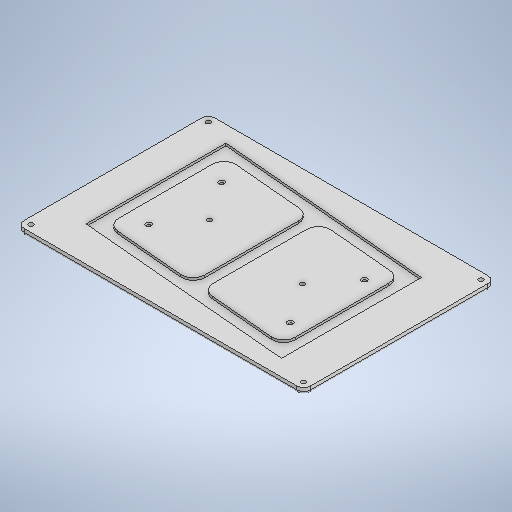
# Autodesk Inventor part: BackPlate
Saved by Autodesk Inventor 2025.2 (Build 292293000, 293)
## iProperties
Created: 2026-02-06
Part Number: BackPlate
Material: Generic
Document SubType Name: Modeling
Designer: Joefi
Density: 1 g/cm^3
Appearance: Default
Mass: 233.651 g
Surface Area: 902.919 cm^2
Volume: 233.651 cm^3
Author: Joefi
Autodesk Inventor part; units mm, degrees
ref_plane "YZ Plane" through (0, 0, 0) normal (1, 0, 0) x (0, 1, 0)
ref_plane "XZ Plane" through (0, 0, 0) normal (0, 1, 0) x (-1, 0, 0)
ref_plane "XY Plane" through (0, 0, 0) normal (0, 0, 1) x (1, 0, 0)
sketch "Sketch1" plane through (0, 0, 0) normal (0, 1, 0) x (-1, 0, 0)
  circle A0 centre (119, 77.3333) radius 2
  circle A1 centre (-119, -77.3333) radius 2
  arc A2 (119, -83.3333) -> (125, -77.3333) centre (119, -77.3333) ccw
  line L0 (125, -77.3333) -> (125, 77.3333)
  arc A3 (125, 77.3333) -> (119, 83.3333) centre (119, 77.3333) ccw
  line L1 (119, 83.3333) -> (-119, 83.3333)
  arc A4 (-119, 83.3333) -> (-125, 77.3333) centre (-119, 77.3333) ccw
  line L2 (-125, 77.3333) -> (-125, -77.3333)
  arc A5 (-125, -77.3333) -> (-119, -83.3333) centre (-119, -77.3333) ccw
  line L3 (-119, -83.3333) -> (119, -83.3333)
  line L4 (119, 71.3333) -> (119, -71.3333)
  arc A6 (119, -71.3333) -> (113, -77.3333) centre (119, -77.3333) ccw
  line L5 (113, -77.3333) -> (-113, -77.3333)
  arc A7 (-113, -77.3333) -> (-119, -71.3333) centre (-119, -77.3333) ccw
  line L6 (-119, -71.3333) -> (-119, 71.3333)
  arc A8 (-119, 71.3333) -> (-113, 77.3333) centre (-119, 77.3333) ccw
  line L7 (-113, 77.3333) -> (113, 77.3333)
  arc A9 (113, 77.3333) -> (119, 71.3333) centre (119, 77.3333) ccw
  circle A10 centre (-119, 77.3333) radius 2
  circle A11 centre (119, -77.3333) radius 2
  point P0 (0, 0)
  point P1 (0, 0)
  dimension "d20" = 4
  dimension "d21" = 4
  dimension "d22" = 4
  dimension "d23" = 4
  constraints: 16 end point, 16 point on circle, 12 centre point, 4 horizontal, 4 vertical, 38 other
  measures "d20" diameter of A1
  measures "d21" diameter of A10
  measures "d22" diameter of A0
  measures "d23" diameter of A11
extrude "Extrusion1" add sketch "Sketch1" along normal blind 6 contours L3 A5 L2 A4 L1 A3 L0 A2 | L4 A6 L5 A7 L6 A8 L7 A9
sketch "Sketch4" plane through (0, 6, 0) normal (0, 1, 0) x (1, 0, 0)
  line L0 (-102.1195, -45.2048) -> (-102.1195, -30.4721) construction
  line L1 (-75.2032, -31.8232) -> (-102.1195, -29.4683) construction
  line L2 (-0.5, -66.4658) -> (-89.7961, -58.6534) construction
  line L3 (-73.7032, -31.4525) -> (-15, -36.5884) construction
  line L4 (-102.1195, -30.4721) -> (-15.8441, -38.0202) construction
  line L5 (-73.7032, 44.3489) -> (-73.7032, -31.4525) construction
  line L6 (-102.1195, -29.4683) -> (-102.1195, 47.3369) construction
  line L7 (-103.1195, 60.7112) -> (-103.1195, -45.2048) construction
  line L8 (-13.5, -39.8412) -> (-13.5, 41.8938) construction
  line L9 (-15, -36.5884) -> (-15, 39.213) construction
  line L10 (-16.1525, 40.8196) -> (-102.1195, 48.3407) construction
  line L11 (-15, 39.213) -> (-73.7032, 44.3489) construction
  line L12 (-13.5, 41.8938) -> (0.1542, 54.4056) construction
  line L13 (-0.5, 55.1624) -> (-16.1525, 40.8196) construction
  line L14 (-87.4429, 74.1598) -> (-0.5, 66.5533) construction
  line L15 (-0.5, 66.5533) -> (-0.5, 55.1624) construction
  line L16 (0.5, 54.7653) -> (0.5, 66.4658) construction
  line L17 (0.1542, 54.4056) -> (13.5, 39.8412) construction
  line L18 (15.8441, 38.0202) -> (0.5, 54.7653) construction
  line L19 (-75.2032, 44.982) -> (-75.2032, -31.8232) construction
  line L20 (0.5, -55.1624) -> (16.1525, -40.8196) construction
  line L21 (0.5, -66.5533) -> (0.5, -55.1624) construction
  line L22 (-0.5, -54.7653) -> (-0.5, -66.4658) construction
  line L23 (13.5, -41.8938) -> (-0.1542, -54.4056) construction
  line L24 (-0.1542, -54.4056) -> (-13.5, -39.8412) construction
  line L25 (-15.8441, -38.0202) -> (-0.5, -54.7653) construction
  line L26 (-89.8832, -59.6496) -> (87.3557, -75.156) construction
  line L27 (89.8832, 59.6496) -> (-87.3557, 75.156) construction
  line L28 (102.1195, 45.2048) -> (102.1195, 30.4721) construction
  arc A0 (102.1195, 45.2048) -> (89.7961, 58.6534) centre (88.6195, 45.2048) ccw construction
  arc A1 (103.1195, 45.2048) -> (89.8832, 59.6496) centre (88.6195, 45.2048) ccw construction
  line L29 (75.2032, 31.8232) -> (102.1195, 29.4683) construction
  line L30 (14.5, -39.6712) -> (14.5, 37.134) construction
  line L31 (13.5, 39.8412) -> (13.5, -41.8938) construction
  line L32 (14.5, 37.134) -> (74.2032, 31.9107) construction
  line L33 (74.2032, -44.8945) -> (14.5, -39.6712) construction
  line L34 (75.2032, -44.982) -> (75.2032, 31.8232) construction
  line L35 (0.5, 66.4658) -> (89.7961, 58.6534) construction
  line L36 (87.4429, -74.1598) -> (0.5, -66.5533) construction
  line L37 (102.1195, 30.4721) -> (15.8441, 38.0202) construction
  line L38 (16.1525, -40.8196) -> (102.1195, -48.3407) construction
  line L39 (103.1195, -60.7112) -> (103.1195, 45.2048) construction
  line L40 (102.1195, -47.3369) -> (75.2032, -44.982) construction
  line L41 (102.1195, -48.3407) -> (102.1195, -60.7112) construction
  arc A2 (87.4429, -74.1598) -> (102.1195, -60.7112) centre (88.6195, -60.7112) ccw construction
  arc A3 (87.3557, -75.156) -> (103.1195, -60.7112) centre (88.6195, -60.7112) ccw construction
  line L42 (102.1195, 29.4683) -> (102.1195, -47.3369) construction
  line L43 (74.2032, 31.9107) -> (74.2032, -44.8945) construction
  arc A4 (-102.1195, -45.2048) -> (-89.7961, -58.6534) centre (-88.6195, -45.2048) ccw construction
  arc A5 (-103.1195, -45.2048) -> (-89.8832, -59.6496) centre (-88.6195, -45.2048) ccw construction
  arc A6 (-87.3557, 75.156) -> (-103.1195, 60.7112) centre (-88.6195, 60.7112) ccw construction
  arc A7 (-87.4429, 74.1598) -> (-102.1195, 60.7112) centre (-88.6195, 60.7112) ccw construction
  line L44 (-102.1195, 48.3407) -> (-102.1195, 60.7112) construction
  line L45 (-102.1195, 47.3369) -> (-75.2032, 44.982) construction
  line L46 (5, -48) -> (-5, -48)
  line L47 (-5, -48) -> (-5, 48)
  line L48 (-5, 48) -> (5, 48)
  line L49 (5, 48) -> (5, -48)
  line L50 (5, -48) -> (-5, 48) construction
  line L51 (-5, -48) -> (5, 48) construction
  line L52 (-90.4115, -45.6034) -> (-90.4115, 61.1094) construction
  line L53 (-90.4115, 63.7374) -> (86.4661, 48.2626) construction
  line L54 (86.4661, 45.2048) -> (86.4661, -60.7112) construction
  line L55 (86.4661, -63.7374) -> (-90.4115, -48.2626) construction
  line L56 (91.4661, -55.7532) -> (86.4661, -55.7532)
  line L57 (81.4661, -55.7532) -> (81.4661, 40.2468)
  line L58 (86.4661, 40.2468) -> (91.4661, 40.2468)
  line L59 (91.4661, 40.2468) -> (91.4661, -55.7532)
  line L60 (91.4661, -55.7532) -> (81.4661, 40.2468) construction
  line L61 (81.4661, -55.7532) -> (91.4661, 40.2468) construction
  line L62 (-90.4115, -40.247) -> (-95.4115, -40.247)
  line L63 (-95.4115, -40.247) -> (-95.4115, 55.753)
  line L64 (-95.4115, 55.753) -> (-90.4115, 55.753)
  line L65 (-85.4115, 55.753) -> (-85.4115, -40.247)
  line L66 (-85.4115, -40.247) -> (-95.4115, 55.753) construction
  line L67 (-95.4115, -40.247) -> (-85.4115, 55.753) construction
  line L68 (95.2186, -69.5222) -> (-100.0356, -52.4397)
  line L69 (-100.0356, -52.4397) -> (-99.164, -42.4778)
  line L70 (96.0902, -59.5603) -> (95.2186, -69.5222)
  line L71 (95.2186, -69.5222) -> (-99.164, -42.4778) construction
  line L72 (-100.0356, -52.4397) -> (96.0902, -59.5603) construction
  line L73 (-100.0356, 59.5603) -> (-99.164, 69.5222)
  line L74 (-99.164, 69.5222) -> (96.0902, 52.4397)
  line L75 (96.0902, 52.4397) -> (95.2186, 42.4778)
  line L76 (95.2186, 42.4778) -> (-99.164, 69.5222) construction
  line L77 (-100.0356, 59.5603) -> (96.0902, 52.4397) construction
  line L78 (81.4661, 40.2468) -> (81.4661, 43.681)
  line L79 (91.4661, -55.7532) -> (91.4661, -59.1557)
  line L80 (5, -48) -> (5, -51.5909)
  line L81 (-5, 48) -> (-5, 51.2458)
  line L82 (-95.4115, 55.753) -> (-95.4115, 59.1557)
  line L83 (-85.4115, -40.247) -> (-85.4115, -43.681)
  line L84 (5, 48) -> (5, 50.3709)
  line L85 (-5, -48) -> (-5, -50.716)
  line L86 (-95.4115, -40.247) -> (-95.4115, -42.8061)
  line L87 (-85.4115, 55.753) -> (-85.4115, 58.2808)
  line L88 (91.4661, 40.2468) -> (91.4661, 42.8061)
  line L89 (81.4661, -55.7532) -> (81.4661, -58.2808)
  line L90 (-90.4115, 58.7183) -> (-100.0356, 59.5603)
  line L91 (-99.164, -42.4778) -> (-90.4115, -43.2435)
  line L92 (86.4661, -58.7183) -> (96.0902, -59.5603)
  line L93 (95.2186, 42.4778) -> (86.4661, 43.2435)
  line L94 (81.4661, 43.681) -> (3.7512, 50.4801)
  line L95 (-3.4428, 51.1095) -> (-85.4115, 58.2808)
  line L96 (-85.4115, -43.681) -> (-3.4074, -50.8554)
  line L97 (3.0989, -51.4246) -> (81.4661, -58.2808)
  line L98 (-95.4115, -42.8061) -> (-95.4115, -52.8443)
  line L99 (-95.4115, 59.1557) -> (-95.4115, 69.1939)
  line L100 (91.4661, 42.8061) -> (91.4661, 52.8443)
  line L101 (91.4661, -59.1557) -> (91.4661, -69.1939)
  point P0 (0, 0)
  point P1 (0, 0)
  point P2 (86.4661, -7.7532)
  point P3 (-90.4115, 7.753)
  point P4 (-1.9727, -56)
  point P5 (-1.9727, 56)
  point P6 (-1.9727, 56)
  dimension "d2" = 10
  dimension "d3" = 96
  dimension "d4" = 10
  dimension "d5" = 96
  dimension "d6" = 10
  dimension "d7" = 96
  dimension "d8" = 10
  dimension "d11" = 196
  dimension "d12" = 10
  dimension "d13" = 196
  dimension "d48" = 56
  dimension "d49" = 56
  constraints: 200 end point, 32 parallel, 25 vertical, 19 point on line, 16 point on circle, 13 midpoint, 8 centre point, 7 perpendicular, 3 horizontal, 112 other
  measures "d2" distance of L47.end L48.end
  measures "d3" distance of L46.end L47.end
  measures "d4" distance of L57.end L58.end
  measures "d5" distance of L57.start L57.end
  measures "d6" distance of L63.end L65.start
  measures "d7" distance of L62.end L63.end
  measures "d8" distance of L68.end L69.end
  measures "d11" distance of L68.start L68.end
  measures "d12" distance of L73.start L73.end
  measures "d13" distance of L73.end L74.end
  measures "d48" vertical distance of point (0, 0) point (-1.973, -56)
  measures "d49" vertical distance of point (-1.973, 56) point (0, 0)
extrude "Extrusion2" cut sketch "Sketch4" against normal blind 2 contours L46 L47 L48 L49 | L59 L79 L101 L68 L98 L86 L63 L82 L99 L74 L100 L88
sketch "Sketch5" plane through (0, 0, 0) normal (0, -1, 0) x (1, 0, 0)
  circle A0 centre (119, 77.3333) radius 2.45
  circle A1 centre (-119, -77.3333) radius 2.45
  arc A2 (119, -83.3333) -> (125, -77.3333) centre (119, -77.3333) ccw
  line L0 (125, -77.3333) -> (125, 77.3333)
  arc A3 (125, 77.3333) -> (119, 83.3333) centre (119, 77.3333) ccw
  line L1 (119, 83.3333) -> (-119, 83.3333)
  arc A4 (-119, 83.3333) -> (-125, 77.3333) centre (-119, 77.3333) ccw
  line L2 (-125, 77.3333) -> (-125, -77.3333)
  arc A5 (-125, -77.3333) -> (-119, -83.3333) centre (-119, -77.3333) ccw
  line L3 (-119, -83.3333) -> (119, -83.3333)
  line L4 (119, 71.3333) -> (119, -71.3333)
  arc A6 (119, -71.3333) -> (113, -77.3333) centre (119, -77.3333) ccw
  line L5 (113, -77.3333) -> (-113, -77.3333)
  arc A7 (-113, -77.3333) -> (-119, -71.3333) centre (-119, -77.3333) ccw
  line L6 (-119, -71.3333) -> (-119, 71.3333)
  arc A8 (-119, 71.3333) -> (-113, 77.3333) centre (-119, 77.3333) ccw
  line L7 (-113, 77.3333) -> (113, 77.3333)
  arc A9 (113, 77.3333) -> (119, 71.3333) centre (119, 77.3333) ccw
  circle A10 centre (-119, 77.3333) radius 2.45
  circle A11 centre (119, -77.3333) radius 2.45
  circle A12 centre (-44.3516, -3.8803) radius 6
  circle A13 centre (44.3516, 3.8803) radius 6
  circle A14 centre (-44.3516, -3.8803) radius 2
  circle A15 centre (44.3516, 3.8803) radius 2
  point P0 (0, 0)
  point P1 (0, 0)
  dimension "d16" = 4
  dimension "d17" = 4
  constraints: 16 centre point, 16 end point, 16 point on circle, 2 coincident
  measures "d16" diameter of A14
  measures "d17" diameter of A15
extrude "Extrusion3" cut sketch "Sketch5" against normal through all contours A14 | A15
chamfer "Chamfer1" distance 1 angle 45 6 edges at (-117, 0, -77.3333) (-46.3516, 0, -3.8803) (-117, 0, 77.3333) (42.3516, 0, 3.8803) (121, 0, 77.3333) (121, 0, -77.3333)
fillet "Fillet1" radius 3 8 edges at (123.2426, 0, -81.576) (0, 0, -83.3333) (-123.2426, 0, -81.576) (-125, 0, 0) (-123.2426, 0, 81.576) (0, 0, 83.3333) (123.2426, 0, 81.576) (125, 0, 0)
sketch "Sketch6" plane through (0, 6, 0) normal (0, 1, 0) x (1, 0, 0)
  arc A0 (-87.3557, 75.156) -> (-103.1195, 60.7112) centre (-88.6195, 60.7112) ccw construction
  arc A1 (-87.4429, 74.1598) -> (-102.1195, 60.7112) centre (-88.6195, 60.7112) ccw construction
  line L0 (-102.1195, 48.3407) -> (-102.1195, 60.7112) construction
  line L1 (-16.1525, 40.8196) -> (-102.1195, 48.3407) construction
  line L2 (-15, 39.213) -> (-73.7032, 44.3489) construction
  line L3 (-87.4429, 74.1598) -> (-0.5, 66.5533) construction
  line L4 (89.8832, 59.6496) -> (-87.3557, 75.156) construction
  line L5 (-0.5, 55.1624) -> (-16.1525, 40.8196) construction
  line L6 (-0.5, 66.5533) -> (-0.5, 55.1624) construction
  line L7 (0.5, 54.7653) -> (0.5, 66.4658) construction
  line L8 (0.1542, 54.4056) -> (13.5, 39.8412) construction
  line L9 (15.8441, 38.0202) -> (0.5, 54.7653) construction
  line L10 (-13.5, 41.8938) -> (0.1542, 54.4056) construction
  line L11 (-0.5, -66.4658) -> (-89.7961, -58.6534) construction
  line L12 (-15.8441, -38.0202) -> (-0.5, -54.7653) construction
  line L13 (-0.1542, -54.4056) -> (-13.5, -39.8412) construction
  line L14 (13.5, -41.8938) -> (-0.1542, -54.4056) construction
  arc A2 (-102.1195, -45.2048) -> (-89.7961, -58.6534) centre (-88.6195, -45.2048) ccw construction
  arc A3 (-103.1195, -45.2048) -> (-89.8832, -59.6496) centre (-88.6195, -45.2048) ccw construction
  line L15 (-0.5, -54.7653) -> (-0.5, -66.4658) construction
  line L16 (0.5, -66.5533) -> (0.5, -55.1624) construction
  line L17 (-89.8832, -59.6496) -> (87.3557, -75.156) construction
  line L18 (0.5, -55.1624) -> (16.1525, -40.8196) construction
  line L19 (14.5, -39.6712) -> (14.5, 37.134) construction
  line L20 (13.5, 39.8412) -> (13.5, -41.8938) construction
  line L21 (74.2032, 31.9107) -> (74.2032, -44.8945) construction
  line L22 (75.2032, -44.982) -> (75.2032, 31.8232) construction
  line L23 (103.1195, -60.7112) -> (103.1195, 45.2048) construction
  line L24 (102.1195, 29.4683) -> (102.1195, -47.3369) construction
  line L25 (102.1195, -47.3369) -> (75.2032, -44.982) construction
  line L26 (74.2032, -44.8945) -> (14.5, -39.6712) construction
  line L27 (16.1525, -40.8196) -> (102.1195, -48.3407) construction
  line L28 (87.4429, -74.1598) -> (0.5, -66.5533) construction
  line L29 (102.1195, -48.3407) -> (102.1195, -60.7112) construction
  line L30 (14.5, 37.134) -> (74.2032, 31.9107) construction
  line L31 (102.1195, 30.4721) -> (15.8441, 38.0202) construction
  line L32 (0.5, 66.4658) -> (89.7961, 58.6534) construction
  line L33 (75.2032, 31.8232) -> (102.1195, 29.4683) construction
  line L34 (102.1195, 45.2048) -> (102.1195, 30.4721) construction
  arc A4 (102.1195, 45.2048) -> (89.7961, 58.6534) centre (88.6195, 45.2048) ccw construction
  arc A5 (103.1195, 45.2048) -> (89.8832, 59.6496) centre (88.6195, 45.2048) ccw construction
  line L35 (-102.1195, -45.2048) -> (-102.1195, -30.4721) construction
  line L36 (-75.2032, -31.8232) -> (-102.1195, -29.4683) construction
  line L37 (-73.7032, -31.4525) -> (-15, -36.5884) construction
  line L38 (-102.1195, -30.4721) -> (-15.8441, -38.0202) construction
  line L39 (-15, -36.5884) -> (-15, 39.213) construction
  line L40 (-13.5, -39.8412) -> (-13.5, 41.8938) construction
  line L41 (-102.1195, 47.3369) -> (-75.2032, 44.982) construction
  line L42 (-75.2032, 44.982) -> (-75.2032, -31.8232) construction
  line L43 (-103.1195, 60.7112) -> (-103.1195, -45.2048) construction
  line L44 (-102.1195, -29.4683) -> (-102.1195, 47.3369) construction
  line L45 (-73.7032, 44.3489) -> (-73.7032, -31.4525) construction
  arc A6 (87.4429, -74.1598) -> (102.1195, -60.7112) centre (88.6195, -60.7112) ccw construction
  arc A7 (87.3557, -75.156) -> (103.1195, -60.7112) centre (88.6195, -60.7112) ccw construction
  circle A8 centre (-67.7032, -25.9545) radius 6
  circle A9 centre (-67.7032, 37.801) radius 6
  circle A10 centre (68.2032, -38.3467) radius 6
  circle A11 centre (68.2032, 26.4127) radius 6
  circle A12 centre (-67.7032, -25.9545) radius 1.45
  circle A13 centre (-67.7032, 37.801) radius 1.45
  circle A14 centre (68.2032, 26.4127) radius 1.45
  circle A15 centre (68.2032, -38.3467) radius 1.45
  point P0 (0, 0)
  point P1 (0, 0)
  point P2 (0, 0)
  point P3 (88.6195, -7.7532)
  point P4 (-88.6195, 7.7532)
  dimension "d38" = 12
  dimension "d39" = 12
  dimension "d40" = 12
  dimension "d41" = 12
  dimension "d42" = 2.9
  constraints: 92 end point, 20 vertical, 16 centre point, 16 point on circle, 8 tangent, 4 coincident, 3 equal radius, 101 other
  measures "d38" diameter of A8
  measures "d39" diameter of A9
  measures "d40" diameter of A10
  measures "d41" diameter of A11
  measures "d42" diameter of A12
extrude "Extrusion4" cut sketch "Sketch6" against normal blind 4 contours A12 | A13 | A14 | A15
chamfer "Chamfer2" distance 1 angle 45 4 edges at (-69.1532, 6, -37.801) (-69.1532, 6, 25.9545) (66.7532, 6, 38.3467) (66.7532, 6, -26.4127)
fillet "Fillet2" radius 10 8 edges at (-5, 5, 50.716) (-5, 5, -51.2458) (5, 5, -50.3709) (81.4661, 5, -43.681) (81.4661, 5, 58.2808) (5, 5, 51.5909) (-85.4115, 5, 43.681) (-85.4115, 5, -58.2808)
equation "\"d13\" = d11"
equation "\"d17\" = d16"
body "Solid1"
